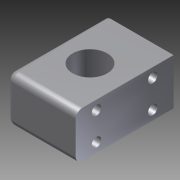
# Autodesk Inventor part: V5 multi bottom
Saved by Autodesk Inventor 2012 (Build 160160000, 160)
## iProperties
Created: 2013-01-29
Part Number: V5 multi bottom
Material: Default
Document SubType Name: Modeling
Designer: mce
Density: 1 g/cm^3
Mass: 20.0127 g
Surface Area: 72.4387 cm^2
Volume: 20.0127 cm^3
Author: mce
Autodesk Inventor part; units mm, degrees
ref_plane "YZ Plane" through (0, 0, 0) normal (1, 0, 0) x (0, 1, 0)
ref_plane "XZ Plane" through (0, 0, 0) normal (0, 1, 0) x (-1, 0, 0)
ref_plane "XY Plane" through (0, 0, 0) normal (0, 0, 1) x (1, 0, 0)
sketch "Sketch1" plane through (0, 0, 0) normal (0, 0, 1) x (1, 0, 0)
  line L0 (0, 0) -> (30, 0)
  line L1 (30, 0) -> (30, 42.4)
  line L2 (30, 42.4) -> (0, 42.4)
  line L3 (0, 42.4) -> (0, 0)
  circle A0 centre (15, 21.2) radius 7.5
  dimension "d0" = 42.4
  dimension "d1" = 30
  dimension "d2" = 15
  dimension "d3" = 21.2
  dimension "d4" = 15
  constraints: 8 end point, 2 horizontal, 2 vertical, 1 centre point
  measures "d0" distance of L2.end L0.start
  measures "d1" distance of L0.start L0.end
  measures "d2" diameter of A0
  measures "d3" distance from line of L2 A0.centre
  measures "d4" distance from line of L3 A0.centre
extrude "Extrusion1" add sketch "Sketch1" along normal blind 20
sketch "Sketch2" plane through (0, 0, 0) normal (-1, 0, 0) x (0, 0, 1)
  line L0 (20, 0) -> (20, 42.4) projected
  line L1 (0, 42.4) -> (20, 42.4) projected
  line L2 (0, 42.4) -> (0, 0) projected
  line L3 (0, 0) -> (20, 0) projected
  circle A0 centre (4, 33.4) radius 2.05
  circle A1 centre (16, 33.4) radius 2.05
  circle A2 centre (4, 9) radius 2.05
  circle A3 centre (16, 9) radius 2.05
  dimension "d7" = 4.1
  dimension "d8" = 4
  dimension "d9" = 4
  dimension "d10" = 4
  dimension "d11" = 4
  dimension "d12" = 9
  dimension "d13" = 9
  dimension "d14" = 9
  dimension "d15" = 9
  constraints: 4 centre point, 3 equal radius
  measures "d7" diameter of A0
  measures "d8" distance from line of L2 A0.centre
  measures "d9" distance from line of L0 A1.centre
  measures "d10" distance from line of L2 A2.centre
  measures "d11" distance from line of L0 A3.centre
  measures "d12" distance from line of L1 A0.centre
  measures "d13" distance from line of L1 A1.centre
  measures "d14" distance from line of L3 A2.centre
  measures "d15" distance from line of L3 A3.centre
extrude "Extrusion6" cut sketch "Sketch2" against normal through all contours A0 | A1 | A2 | A3
fillet "Fillet3" radius 3 3 edges at (0, 21.2, 20) (0, 21.2, 0) (0, 0, 10)
fillet "Fillet4" radius 3 4 edges at (0.8787, 0.8787, 19.1213) (16.5, 0, 20) (0.8787, 0.8787, 0.8787) (16.5, 0, 0)
sketch "Sketch3" plane through (0, 0, 0) normal (0, -1, 0) x (1, 0, 0)
  line L0 (30, 20) -> (0, 20) projected
  line L1 (0, 0) -> (0, 20) projected
  line L2 (30, 0) -> (30, 20) projected
  circle A0 centre (5, 10) radius 2.05
  circle A1 centre (25, 10) radius 2.05
  dimension "d18" = 4.1
  dimension "d19" = 5
  dimension "d20" = 5
  dimension "d21" = 10
  dimension "d22" = 10
  constraints: 2 centre point, 1 equal radius
  measures "d18" diameter of A0
  measures "d19" distance from line of L1 A0.centre
  measures "d20" distance from line of L2 A1.centre
  measures "d21" distance from line of L0 A0.centre
  measures "d22" distance from line of L0 A1.centre
sketch "Sketch4" plane through (0, 0, 0) normal (-1, 0, 0) x (0, 0, 1)
  circle A0 centre (16, 9) radius 2.05 projected
  circle A1 centre (4, 9) radius 2.05 projected
  circle A2 centre (16, 33.4) radius 2.05 projected
  circle A3 centre (4, 33.4) radius 2.05 projected
  circle A4 centre (4, 33.4) radius 3.75
  circle A5 centre (16, 33.4) radius 3.75
  circle A6 centre (4, 9) radius 3.75
  circle A7 centre (16, 9) radius 3.75
  dimension "d25" = 7.5
  constraints: 4 centre point, 4 coincident, 3 equal radius
  measures "d25" diameter of A4
sketch "Sketch5" plane through (0, 0, 0) normal (0, -1, 0) x (1, 0, 0)
  circle A0 centre (25, 10) radius 2.05 projected
  circle A1 centre (5, 10) radius 2.05 projected
  circle A2 centre (5, 10) radius 3.75
  circle A3 centre (25, 10) radius 3.75
  dimension "d28" = 7.5
  constraints: 2 centre point, 2 coincident, 1 equal radius
  measures "d28" diameter of A2
equation "\"d3\" = 0.5 * d0"
equation "\"d9\" = d8"
equation "\"d10\" = d8"
equation "\"d11\" = d8"
equation "\"d13\" = d12"
equation "\"d14\" = d12"
equation "\"d15\" = d12"
equation "\"d20\" = d19"
body "Solid1"
